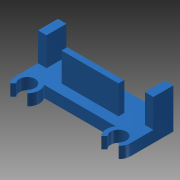
# Autodesk Inventor part: switch lever
Saved by Autodesk Inventor 2013 (Build 170138000, 138)
## iProperties
Created: 2017-02-13
Part Number: switch lever
Material: Generic
Document SubType Name: Modeling
Designer: Herman de Vries
Density: 1 g/cm^3
Author: Herman de Vries
Autodesk Inventor part; units mm, degrees
ref_plane "YZ Plane" through (0, 0, 0) normal (1, 0, 0) x (0, 1, 0)
ref_plane "XZ Plane" through (0, 0, 0) normal (0, 1, 0) x (-1, 0, 0)
ref_plane "XY Plane" through (0, 0, 0) normal (0, 0, 1) x (1, 0, 0)
sketch "Sketch1" plane through (0, 0, 0) normal (0, 0, 1) x (1, 0, 0)
  line L0 (0, 0) -> (32, 0) construction
  line L1 (32, 0) -> (32, 15) construction
  line L2 (32, 15) -> (0, 15) construction
  line L3 (0, 15) -> (0, 0) construction
  circle A0 centre (0, 0) radius 2.75
  circle A1 centre (32, 0) radius 2.75
  line L4 (16, 15) -> (16, 0)
  line L5 (36.25, 0) -> (36.25, 15)
  line L6 (36.25, 15) -> (-4.25, 15)
  line L7 (-4.25, 15) -> (-4.25, 0)
  circle A2 centre (0, 0) radius 4.25
  circle A3 centre (32, 0) radius 4.25
  line L8 (3.4369, 2.5) -> (28.5631, 2.5)
  point P0 (0, 4.25)
  point P1 (32, 4.25)
  dimension "d0" = 32
  dimension "d2" = 15
  dimension "d4" = 5.5
  dimension "d6" = 1.5
  dimension "d7" = 1.5
  dimension "d10" = 5.5
  dimension "d11" = 2.5
  constraints: 18 end point, 6 point on circle, 5 coincident, 4 centre point, 3 parallel, 3 point on line, 2 midpoint, 2 perpendicular, 2 tangent, 1 collinear, 1 horizontal, 1 vertical
  measures "d0" distance of L1.end L2.end
  measures "d2" distance of L2.end L0.start
  measures "d4" diameter of A1
  measures "d6" radial gap between concentric circles of A2 A0
  measures "d7" radial gap between concentric circles of A3 A1
  measures "d10" diameter of A0
  measures "d11" distance between parallel lines of L0 L8
extrude "Extrusion1" add sketch "Sketch1" along normal blind 4
sketch "Sketch2" plane through (0, 0, 4) normal (0, 0, 1) x (1, 0, 0)
  line L0 (-4.25, 15) -> (-4.25, 0) projected
  line L1 (3.4369, 2.5) -> (28.5631, 2.5) projected
  line L2 (36.25, 0) -> (36.25, 15) projected
  line L3 (0, 0) -> (-4.0526, -4.0526)
  line L4 (-4.0526, -4.0526) -> (0.938, -9.0431)
  line L5 (0.938, -9.0431) -> (4.9905, -4.9905)
  line L6 (4.9905, -4.9905) -> (0, 0)
  circle A0 centre (32, 0) radius 2.75 construction
  line L7 (32, 0) -> (27.2846, -4.7154)
  line L8 (27.2846, -4.7154) -> (32.2729, -9.7038)
  line L9 (32.2729, -9.7038) -> (36.9883, -4.9883)
  line L10 (36.9883, -4.9883) -> (32, 0)
  dimension "d24" = 45
  constraints: 16 end point, 4 parallel, 3 perpendicular
  measures "d24" angle of L1 L6
extrude "Extrusion2" cut sketch "Sketch2" against normal through all
sketch "Sketch3" plane through (0, 0, 4) normal (0, 0, 1) x (1, 0, 0)
  line L0 (-4.25, 15) -> (-1.25, 15)
  line L1 (-1.25, 15) -> (-1.25, 8)
  line L2 (-1.25, 8) -> (-4.25, 8)
  line L3 (-4.25, 8) -> (-4.25, 15)
  line L4 (36.25, 15) -> (33.25, 15)
  line L5 (33.25, 15) -> (33.25, 8)
  line L6 (33.25, 8) -> (36.25, 8)
  line L7 (36.25, 8) -> (36.25, 15)
  line L8 (6, 6) -> (26, 6)
  line L9 (26, 6) -> (26, 8)
  line L10 (26, 8) -> (6, 8)
  line L11 (6, 8) -> (6, 6)
  line L12 (3.4369, 2.5) -> (28.5631, 2.5) projected
  point P0 (0, 0)
  point P1 (16, 6)
  point P2 (16, 2.5)
  dimension "d18" = 3
  dimension "d19" = 7
  dimension "d20" = 3
  dimension "d21" = 7
  dimension "d25" = 2
  dimension "d26" = 20
  constraints: 24 end point, 6 parallel, 3 horizontal, 3 perpendicular, 2 midpoint, 1 collinear, 1 vertical alignment
  measures "d18" distance of L1.end L2.end
  measures "d19" distance of L0.end L1.end
  measures "d20" distance of L5.end L6.end
  measures "d21" distance of L6.end L4.start
  measures "d25" distance of L9.end L8.end
  measures "d26" distance of L8.start L8.end
extrude "Extrusion3" add sketch "Sketch3" along normal blind 10
equation "\"d4\" = d10"
equation "\"d7\" = d6"
equation "\"d20\" = d18"
equation "\"d21\" = d19"
body "Solid1"
